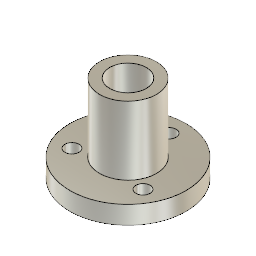
_lead screw nut mock.514bb80c-a6ec-4590-85a8-551880e0ad4e (Autodesk Fusion 360 design; units mm, degrees)
Autodesk Fusion 360 part; units mm, degrees
sketch "Sketch1" plane through (0, 0, 0) normal (0, 0, 1) x (1, 0, 0)
  circle A0 centre (0, 0) radius 12.75
  circle A1 centre (0, 9) radius 1.55
  circle A2 centre (-7.7942, -4.5) radius 1.55
  circle A3 centre (7.7942, -4.5) radius 1.55
  dimension "d1" = 25.5
  dimension "d2" = 3.1
  dimension "d3" = 9
  dimension "d5" = 360
  measures "d1" diameter of A0
  measures "d2" diameter of A1
  measures "d3" distance of A0.centre
extrude "Extrude1" add sketch "Sketch1" along normal blind 4
sketch "Sketch2" plane through (0, 0, 4) normal (0, 0, 1) x (-1, 0, 0)
  circle A0 centre (-7.7942, 4.5) radius 1.55
  circle A1 centre (7.7942, 4.5) radius 1.55
  circle A2 centre (0, -9) radius 1.55
  circle A3 centre (0, 0) radius 12.75
  circle A4 centre (0, 0) radius 6.25
  circle A5 centre (0, 0) radius 4
  dimension "d8" = 12.5
  dimension "d9" = 8
  measures "d8" diameter of A4
  measures "d9" diameter of A5
extrude "Extrude2" add sketch "Sketch2" along normal blind 15 contours A4
extrude "Extrude3" cut 1 faces at (-0.9485, -1.8197, 4) along direction (0, 0, -1) blind 7
